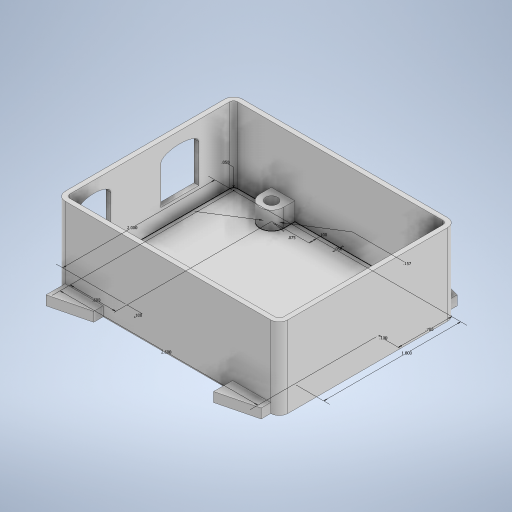
# Autodesk Inventor part: ArduinoHolder-v1
Saved by Autodesk Inventor 2023 (Build 270158030, 158C)
## iProperties
Created: 2024-03-14
Part Number: ArduinoHolder-v1
Material: Generic
Document SubType Name: Modeling
Designer: lvrectanus0
Density: 1 g/cm^3
Appearance: Default
Author: lvrectanus0
Autodesk Inventor part; units mm, degrees
ref_plane "YZ Plane" through (0, 0, 0) normal (1, 0, 0) x (0, 1, 0)
ref_plane "XZ Plane" through (0, 0, 0) normal (0, 1, 0) x (-1, 0, 0)
ref_plane "XY Plane" through (0, 0, 0) normal (0, 0, 1) x (1, 0, 0)
sketch "Sketch1" plane through (0, 0, 0) normal (0, 1, 0) x (-1, 0, 0)
  circle A0 centre (-15.24, 2.54) radius 2
  circle A1 centre (-66.04, 17.78) radius 2
  circle A2 centre (-66.04, 45.72) radius 2
  circle A3 centre (-15.24, 50.8) radius 2
  line L0 (0, 0) -> (-68.58, 0) construction
  line L1 (-68.58, 0) -> (-68.58, 53.34) construction
  line L2 (-68.58, 53.34) -> (0, 53.34) construction
  line L3 (0, 53.34) -> (0, 0) construction
  line L4 (-68.58, -1.27) -> (0, -1.27)
  line L5 (1.27, 0) -> (1.27, 53.34)
  line L6 (0, 54.61) -> (-68.58, 54.61)
  line L7 (-69.85, 53.34) -> (-69.85, 0)
  arc A4 (0, -1.27) -> (1.27, 0) centre (0, 0) ccw
  arc A5 (-69.85, 0) -> (-68.58, -1.27) centre (-68.58, 0) ccw
  arc A6 (-68.58, 54.61) -> (-69.85, 53.34) centre (-68.58, 53.34) ccw
  arc A7 (1.27, 53.34) -> (0, 54.61) centre (0, 53.34) ccw
  arc A8 (-11.335, 2.54) -> (-19.145, 2.54) centre (-15.24, 2.54) ccw
  arc A9 (-19.145, 50.8) -> (-11.335, 50.8) centre (-15.24, 50.8) ccw
  arc A10 (-66.04, 41.815) -> (-66.04, 49.625) centre (-66.04, 45.72) ccw
  arc A11 (-66.04, 13.875) -> (-66.04, 21.685) centre (-66.04, 17.78) ccw
  line L8 (-11.335, 2.54) -> (-19.145, 2.54) construction
  line L9 (-19.145, 2.54) -> (-19.145, -1.27)
  line L10 (-19.145, -1.27) -> (-11.335, -1.27)
  line L11 (-11.335, -1.27) -> (-11.335, 2.54)
  line L12 (-66.04, 13.875) -> (-69.85, 13.875)
  line L13 (-69.85, 13.875) -> (-69.85, 21.685)
  line L14 (-69.85, 21.685) -> (-66.04, 21.685)
  line L15 (-66.04, 21.685) -> (-66.04, 13.875) construction
  line L16 (-66.04, 41.815) -> (-69.85, 41.815)
  line L17 (-69.85, 41.815) -> (-69.85, 49.625)
  line L18 (-69.85, 49.625) -> (-66.04, 49.625)
  line L19 (-66.04, 49.625) -> (-66.04, 41.815) construction
  line L20 (-19.145, 50.8) -> (-11.335, 50.8) construction
  line L21 (-11.335, 50.8) -> (-11.335, 54.61)
  line L22 (-11.335, 54.61) -> (-19.145, 54.61)
  line L23 (-19.145, 54.61) -> (-19.145, 50.8)
  dimension "d0" = 4
  dimension "d4" = 15.24
  dimension "d5" = 2.54
  dimension "d6" = 17.78
  dimension "d7" = 66.04
  dimension "d8" = 45.72
  dimension "d9" = 50.8
  dimension "d10" = 2.54
  dimension "d11" = 2.54
  dimension "d12" = 1.27
  dimension "d13" = 1.27
  dimension "d14" = 1.905
  constraints: 48 end point, 16 point on circle, 13 tangent, 12 centre point, 12 parallel, 9 equal radius, 7 point on line, 6 perpendicular, 5 horizontal, 2 vertical alignment, 3 other
  measures "d0" diameter of A0
  measures "d4" horizontal distance of A0.centre L0.start
  measures "d5" vertical distance of A0.centre L0.start
  measures "d6" vertical distance of A1.centre L0.start
  measures "d7" horizontal distance of L0.start A1.centre
  measures "d8" vertical distance of L0.start A2.centre
  measures "d9" vertical distance of A3.centre L0.start
  measures "d10" distance from line of L1 A1.centre
  measures "d11" distance from line of L2 A3.centre
  measures "d12" distance between parallel lines of L0 L4
  measures "d13" radius of A4
  measures "d14" radial gap between concentric circles of A0 A8
extrude "Extrusion1" add sketch "Sketch1" along normal blind 6 contours L9 A8 L11 L4 | L7 L14 A11 L12 | L7 L18 A10 L16 | L21 A9 L23 L6
extrude "Extrusion2" add sketch "Sketch1" against normal blind 2 contours A0 | A1 | A2 | A3 | A5 L7 L12 A11 L14 L16 A10 L18 A6 L6 L23 A9 L21 A7 L5 A4 L4 L11 A8 L9 | L9 A8 L11 L4 | L7 L14 A11 L12 | L7 L18 A10 L16 | L21 A9 L23 L6
sketch "Sketch2" plane through (0, -2, 0) normal (0, -1, 0) x (1, 0, 0)
  line L0 (68.58, 54.61) -> (0, 54.61) projected
  arc A0 (0, 54.61) -> (-1.27, 53.34) centre (0, 53.34) ccw projected
  line L1 (-1.27, 53.34) -> (-1.27, 0) projected
  arc A1 (-1.27, 0) -> (0, -1.27) centre (0, 0) ccw projected
  line L2 (0, -1.27) -> (68.58, -1.27) projected
  arc A2 (68.58, -1.27) -> (69.85, 0) centre (68.58, 0) ccw projected
  line L3 (69.85, 0) -> (69.85, 53.34) projected
  arc A3 (69.85, 53.34) -> (68.58, 54.61) centre (68.58, 53.34) ccw projected
  line L4 (68.58, -2.8575) -> (0, -2.8575)
  arc A4 (-2.8575, 0) -> (0, -2.8575) centre (0, 0) ccw
  line L5 (-2.8575, 0) -> (-2.8575, 53.34)
  arc A5 (0, 56.1975) -> (-2.8575, 53.34) centre (0, 53.34) ccw
  line L6 (0, 56.1975) -> (68.58, 56.1975)
  arc A6 (71.4375, 53.34) -> (68.58, 56.1975) centre (68.58, 53.34) ccw
  line L7 (71.4375, 53.34) -> (71.4375, 0)
  arc A7 (68.58, -2.8575) -> (71.4375, 0) centre (68.58, 0) ccw
  point P0 (0, 0)
  dimension "d19" = 1.5875
  constraints: 8 end point, 8 point on circle, 4 centre point, 7 other
  measures "d19" distance between parallel lines of L2 L4
extrude "Extrusion3" add sketch "Sketch2" against normal blind 27.05
sketch "Sketch4" plane through (-2.8575, -2, 0) normal (-1, 0, 0) x (0, 0, 1)
  line L0 (2.54, 8) -> (-1.27, 8) projected
  line L1 (-1.27, 8) -> (2.54, 8) projected
  line L2 (2.54, 8) -> (2.54, 8) projected
  line L3 (0.54, 8) -> (4.54, 8) projected
  line L4 (0, 2) -> (53.34, 2) projected
  line L5 (50.8, 8) -> (54.61, 8) projected
  line L6 (54.61, 8) -> (50.8, 8) projected
  line L7 (50.8, 8) -> (50.8, 8) projected
  line L8 (48.8, 8) -> (52.8, 8) projected
  line L9 (0, 27.05) -> (53.34, 27.05) projected
  line L10 (50.8, 8) -> (54.61, 8) projected
  line L11 (50.8, 8) -> (46.895, 8) projected
  line L12 (50.8, 8) -> (50.8, 20.7)
  line L13 (50.8, 20.7) -> (39.6875, 20.7) construction
  line L14 (43.72, 8) -> (47.72, 8) projected
  line L15 (39.6875, 20.7) -> (39.6875, 8)
  line L16 (39.6875, 8) -> (50.8, 8)
  ellipse E0 centre (45.2438, 20.7) end of major axis (50.8, 20.7) minor radius 2.54 (50.8, 20.7) -> (39.6875, 20.7) ccw
  ellipse E1 centre (45.2438, 20.7) end of major axis (50.8, 20.7) minor radius 2.54 (39.6875, 20.7) -> (50.8, 20.7) ccw construction
  line L17 (10.3188, 8) -> (10.3188, 20.7)
  line L18 (10.3188, 8) -> (23.0188, 8)
  line L19 (15.78, 8) -> (19.78, 8) projected
  line L20 (23.0188, 8) -> (23.0188, 20.7)
  ellipse E2 centre (16.6688, 20.7) end of major axis (23.0188, 20.7) minor radius 2.54 (23.0188, 20.7) -> (10.3188, 20.7) ccw
  point P0 (2.54, 2)
  point P1 (2.54, 2)
  point P2 (2.54, 2)
  point P3 (50.8, 2)
  point P4 (2.54, 2)
  point P5 (16.6688, 8)
  dimension "d26" = 2.54
  dimension "d29" = 2.54
  dimension "d24" = 12.7
  dimension "d25" = 11.1125
  dimension "d27" = 10.3187
  dimension "d28" = 12.7
  constraints: 14 end point, 4 vertical, 3 collinear, 3 parallel, 2 midpoint, 1 coincident, 1 horizontal, 1 perpendicular, 1 vertical alignment, 12 other
  measures "d24" distance of L5.start L12.end
  measures "d25" distance of L12.end L13.end
  measures "d27" horizontal distance of L17.start L4.start
  measures "d28" distance of L17.start L18.end
extrude "Extrusion5" cut sketch "Sketch4" against normal up to surface (1.5875 mm away)
sketch "Sketch5" plane through (0, -2, 0) normal (0, -1, 0) x (1, 0, 0)
  line L0 (68.58, 56.1975) -> (0, 56.1975) projected
  arc A0 (0, 56.1975) -> (-2.8575, 53.34) centre (0, 53.34) ccw projected
  line L1 (-2.8575, 53.34) -> (-2.8575, 0) projected
  arc A1 (-2.8575, 0) -> (0, -2.8575) centre (0, 0) ccw projected
  line L2 (0, -2.8575) -> (68.58, -2.8575) projected
  arc A2 (68.58, -2.8575) -> (71.4375, 0) centre (68.58, 0) ccw projected
  line L3 (71.4375, 0) -> (71.4375, 53.34) projected
  arc A3 (71.4375, 53.34) -> (68.58, 56.1975) centre (68.58, 53.34) ccw projected
  line L4 (0, 56.1975) -> (68.58, 56.1975) projected
  line L5 (0, 56.1975) -> (12.7, 56.1975)
  line L6 (12.7, 56.1975) -> (12.7, 59.3725)
  line L7 (0, 62.5475) -> (0, 62.5475)
  line L8 (0, 62.5475) -> (0, 56.1975)
  line L9 (68.58, 56.1975) -> (55.88, 56.1975)
  line L10 (55.88, 56.1975) -> (55.88, 62.5475)
  line L11 (55.88, 62.5475) -> (55.88, 62.5475)
  line L12 (68.58, 59.3725) -> (68.58, 56.1975)
  line L13 (0, -2.8575) -> (12.7, -2.8575)
  line L14 (12.7, -2.8575) -> (12.7, -6.0325)
  line L15 (0, -9.2075) -> (0, -9.2075)
  line L16 (0, -9.2075) -> (0, -2.8575)
  line L17 (68.58, -2.8575) -> (0, -2.8575) projected
  line L18 (68.58, -2.8575) -> (55.88, -2.8575)
  line L19 (55.88, -2.8575) -> (55.88, -9.2075)
  line L20 (55.88, -9.2075) -> (55.88, -9.2075)
  line L21 (68.58, -6.0325) -> (68.58, -2.8575)
  line L22 (12.7, 59.3725) -> (0, 62.5475)
  line L23 (55.88, 62.5475) -> (68.58, 59.3725)
  line L24 (12.7, -6.0325) -> (0, -9.2075)
  line L25 (55.88, -9.2075) -> (68.58, -6.0325)
  point P0 (0, 0)
  point P1 (12.7, 62.5475)
  point P2 (68.58, 62.5475)
  point P3 (12.7, -9.2075)
  point P4 (68.58, -9.2075)
  dimension "d32" = 12.7
  dimension "d33" = 6.35
  dimension "d34" = 12.7
  dimension "d35" = 6.35
  dimension "d36" = 12.7
  dimension "d37" = 6.35
  dimension "d38" = 12.7
  dimension "d39" = 6.35
  dimension "d40" = 3.175
  dimension "d41" = 12.7
  dimension "d42" = 12.7
  dimension "d43" = 3.175
  dimension "d44" = 3.175
  dimension "d45" = 12.7
  dimension "d46" = 12.7
  dimension "d47" = 3.175
  constraints: 40 end point, 8 parallel, 8 point on line, 4 horizontal, 4 perpendicular
  measures "d32" distance of L7.end point (12.7, 62.548)
  measures "d33" distance of point (12.7, 62.548) L5.end
  measures "d34" distance of L10.end point (68.58, 62.547)
  measures "d35" distance of L9.end L10.end
  measures "d36" distance of point (12.7, -9.207) L15.end
  measures "d37" distance of L13.end point (12.7, -9.207)
  measures "d38" distance of point (68.58, -9.208) L19.end
  measures "d39" distance of L19.end L18.end
  measures "d40" distance of L6.end point (12.7, 62.548)
  measures "d41" distance of L7.start point (12.7, 62.548)
  measures "d42" distance of L11.end point (68.58, 62.547)
  measures "d43" distance of L12.start point (68.58, 62.547)
  measures "d44" distance of L14.end point (12.7, -9.207)
  measures "d45" distance of L15.start point (12.7, -9.207)
  measures "d46" distance of L20.end point (68.58, -9.208)
  measures "d47" distance of L21.start point (68.58, -9.208)
extrude "Extrusion6" add sketch "Sketch5" against normal blind 3.175 contours L0 L10 L23 L12 | L0 L8 L22 L6 | L21 L25 L19 L2 | L14 L24 L16 L2
equation "\"d42\" = d41"
equation "\"d43\" = d40"
equation "\"d44\" = d40"
equation "\"d45\" = d41"
equation "\"d46\" = d41"
equation "\"d47\" = d40"
body "Solid1"
